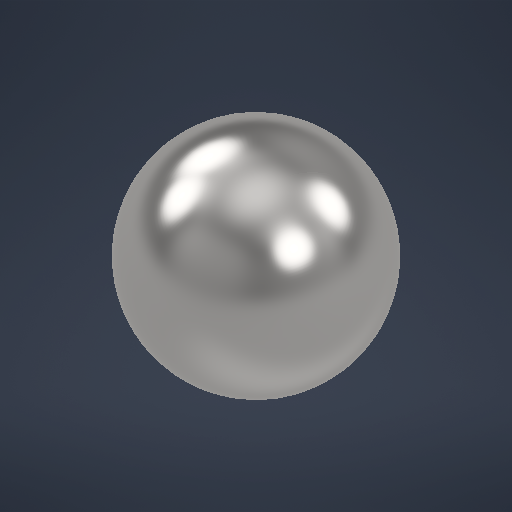
# Autodesk Inventor part: kula_d4mm
Saved by Autodesk Inventor 2026.1 (Build 301233020, 233B)
## iProperties
Created: 2025-11-03
Part Number: kula_d4mm
Material: Stainless Steel
Document SubType Name: Modeling
Designer: Jan
Density: 8 g/cm^3
Appearance: Semi-Polished
Author: Jan
Autodesk Inventor part; units mm, degrees
ref_plane "YZ Plane" through (0, 0, 0) normal (1, 0, 0) x (0, 1, 0)
ref_plane "XZ Plane" through (0, 0, 0) normal (0, 1, 0) x (-1, 0, 0)
ref_plane "XY Plane" through (0, 0, 0) normal (0, 0, 1) x (1, 0, 0)
sketch "Sketch1" plane through (0, 0, 0) normal (0, 1, 0) x (-1, 0, 0)
  circle A0 centre (0, 0) radius 2
  line L0 (2, 0) -> (-2, 0)
  dimension "d0" = 4
  constraints: 2 end point, 2 point on circle, 1 centre point, 1 coincident, 1 horizontal
  measures "d0" diameter of A0
revolve "Revolution1" add sketch "Sketch1" angle 360 about axis through (-2, 0, 0) along (1, 0, 0) picked at (-0.5903, -0.3098) contours A0 L0
body "Solid1"
